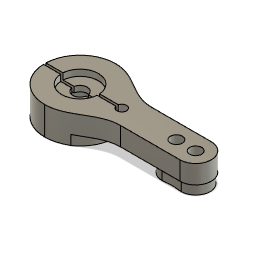
assembled new design (Autodesk Fusion 360 archive; units mm, degrees)
design "servo connector"
Autodesk Fusion 360 part; units mm, degrees
sketch "Sketch1" plane through (0, 0, 0) normal (0, 1, 0) x (1, 0, 0)
  circle A0 centre (0, 0) radius 7.35
  line L0 (0, -3.25) -> (24, -3.25)
  arc A1 (24, -3.25) -> (24, 3.25) centre (24, 0) ccw
  line L1 (24, 3.25) -> (0, 3.25)
  arc A2 (0, 3.25) -> (0, -3.25) centre (0, 0) ccw
  line L2 (0, 0) -> (24, 0) construction
  line L3 (-7.35, 0) -> (11.65, 0) construction
  line L4 (11.65, 0) -> (11.65, 3.25) construction
  circle A3 centre (24, 0) radius 1.25
  circle A4 centre (20, 0) radius 1.25
  spline S0 degree 5 poles (11.65, 3.25) (11.1355, 3.25) (10.1313, 3.3337) (8.6992, 3.7102) (6.9088, 4.6153) (4.7412, 5.9847) (2.9508, 6.8898) (1.5187, 7.2663) (0.5145, 7.35) (0, 7.35) knots 0 0 0 0 0 0 0.2 0.4 0.6 0.8 1 1 1 1 1 1
  line L5 (0, 7.35) -> (0, 0) construction
  spline S1 degree 5 poles (11.65, -3.25) (11.1355, -3.25) (10.1313, -3.3337) (8.6992, -3.7102) (6.9088, -4.6153) (4.7412, -5.9847) (2.9508, -6.8898) (1.5187, -7.2663) (0.5145, -7.35) (0, -7.35) knots 0 0 0 0 0 0 0.2 0.4 0.6 0.8 1 1 1 1 1 1
  line L6 (12.9681, 3.25) -> (10.3319, 3.25)
  line L7 (1.3181, 7.35) -> (-1.3181, 7.35)
  line L8 (12.9681, -3.25) -> (10.3319, -3.25)
  line L9 (1.3181, -7.35) -> (-1.3181, -7.35)
  circle A5 centre (0, 0) radius 1.5
  line L10 (-7.35, 0) -> (8.65, 0) construction
  circle A6 centre (8.65, 0) radius 1
  line L11 (8.65, 0.25) -> (-8, 0.25)
  arc A7 (-8, 0.25) -> (-8, -0.25) centre (-8, 0) ccw
  line L12 (-8, -0.25) -> (8.65, -0.25)
  arc A8 (8.65, -0.25) -> (8.65, 0.25) centre (8.65, 0) ccw
  line L13 (8.65, 0) -> (-8, 0) construction
  dimension "d1" = 14.7
  dimension "d4" = 24
  dimension "d5" = 6.5
  dimension "d6" = 19
  dimension "d7" = 4
  dimension "d8" = 2.5
  dimension "d9" = 2.5
  dimension "d10" = 3
  dimension "d11" = 16
  dimension "d12" = 2
  dimension "d15" = 0.5
  constraint coincident A0.centre A2.centre
  constraint tangent L0 A1
  constraint tangent A1 L1
  constraint parallel L0 L1
  constraint tangent L1 A2
  constraint tangent L0 A2
  constraint horizontal L2
  constraint coincident A0 L3.start
  constraint parallel L2 L3
  constraint coincident L1 L4.end
  constraint perpendicular L1 L4
  constraint concentric A1 A3
  constraint coincident L2 A4.centre
  constraint coincident A0 S0.end
  constraint perpendicular L3 L5
  constraint coincident S0.end L5.start
  constraint tangent A0 S0
  constraint midpoint L4.end L6
  constraint midpoint S0.end L7
  constraint symmetric L3 L4.end S1.start
  constraint symmetric L3 S0.end S1.end
  constraint symmetric L3 L6.start L8.start
  constraint symmetric L3 L6.end L8.end
  constraint symmetric L3 L7.start L9.start
  constraint symmetric L3 L7.end L9.end
  constraint perpendicular L4 L10
  constraint coincident L10.end A6.centre
  constraint tangent L11 A7
  constraint tangent A7 L12
  constraint parallel L11 L12
  constraint tangent L12 A8
  constraint tangent L11 A8
  constraint parallel L3 L13
  measures "d1" diameter of A0
  measures "d4" distance of A0.centre A1.centre
  measures "d5" diameter of A1
  measures "d6" distance of L3.start L3.end
  measures "d7" distance of A1.centre A4.centre
  measures "d8" diameter of A4
  measures "d9" diameter of A3
  measures "d10" diameter of A5
  measures "d11" distance of L3.start L10.end
  measures "d12" diameter of A6
  measures "d15" diameter of A7
extrude "Extrude1" add sketch "Sketch1" along normal blind 5.85 contours A0 L1 A2 A5 L11 | A0 L0 A1 L1 L6 L8 A6 L11 L12 | A0 L0 A2 A5 L12 | A0 L0 A2 L12 | A0 L1 A2 L11 | A0 L1 S0 L6 | A0 L0 S1 L8
sketch "Sketch2" plane through (0, 5.85, 0) normal (0, 1, 0) x (-1, 0, 0)
  circle A0 centre (-20, 0) radius 1.25
  circle A1 centre (-24, 0) radius 1.25
  line L0 (1.479, 0.25) -> (7.3457, 0.25)
  arc A2 (7.3457, 0.25) -> (0, 7.35) centre (0, 0) ccw
  spline S0 degree 5 poles (0, 7.35) (-0.5145, 7.35) (-1.5187, 7.2663) (-2.9508, 6.8898) (-4.7412, 5.9847) (-6.9088, 4.6153) (-8.6992, 3.7102) (-10.1313, 3.3337) (-11.1355, 3.25) (-11.65, 3.25) knots -1 -1 -1 -1 -1 -1 -0.8 -0.6 -0.4 -0.2 0 0 0 0 0 0
  line L1 (-11.65, 3.25) -> (-24, 3.25)
  arc A3 (-24, 3.25) -> (-24, -3.25) centre (-24, 0) ccw
  line L2 (-24, -3.25) -> (-11.65, -3.25)
  spline S1 degree 5 poles (-11.65, -3.25) (-11.1355, -3.25) (-10.1313, -3.3337) (-8.6992, -3.7102) (-6.9088, -4.6153) (-4.7412, -5.9847) (-2.9508, -6.8898) (-1.5187, -7.2663) (-0.5145, -7.35) (0, -7.35) knots 0 0 0 0 0 0 0.2 0.4 0.6 0.8 1 1 1 1 1 1
  arc A4 (0, -7.35) -> (7.3457, -0.25) centre (0, 0) ccw
  line L3 (7.3457, -0.25) -> (1.479, -0.25)
  arc A5 (-1.479, -0.25) -> (1.479, -0.25) centre (0, 0) ccw
  line L4 (-1.479, -0.25) -> (-7.6818, -0.25)
  arc A6 (-7.6818, 0.25) -> (-7.6818, -0.25) centre (-8.65, 0) ccw
  line L5 (-7.6818, 0.25) -> (-1.479, 0.25)
  arc A7 (1.479, 0.25) -> (-1.479, 0.25) centre (0, 0) ccw
  circle A8 centre (0, 0) radius 3.8
  dimension "d16" = 7.6
  constraint concentric A2 A8
  measures "d16" diameter of A8
extrude "Extrude2" cut sketch "Sketch2" against normal blind 1.3 contours L0 L5 A7 A8 | L3 A5 L4 A8
sketch "Sketch3" plane through (0, 0, 0) normal (0, -1, 0) x (1, 0, 0)
  circle A0 centre (20, 0) radius 1.25
  circle A1 centre (24, 0) radius 1.25
  line L0 (-7.3457, 0.25) -> (-1.479, 0.25)
  arc A2 (1.479, 0.25) -> (-1.479, 0.25) centre (0, 0) ccw
  line L1 (1.479, 0.25) -> (7.6818, 0.25)
  arc A3 (7.6818, -0.25) -> (7.6818, 0.25) centre (8.65, 0) ccw
  line L2 (7.6818, -0.25) -> (1.479, -0.25)
  arc A4 (-1.479, -0.25) -> (1.479, -0.25) centre (0, 0) ccw
  line L3 (-1.479, -0.25) -> (-7.3457, -0.25)
  arc A5 (-7.3457, -0.25) -> (0, -7.35) centre (0, 0) ccw
  spline S0 degree 5 poles (11.65, -3.25) (11.1355, -3.25) (10.1313, -3.3337) (8.6992, -3.7102) (6.9088, -4.6153) (4.7412, -5.9847) (2.9508, -6.8898) (1.5187, -7.2663) (0.5145, -7.35) (0, -7.35) knots 0 0 0 0 0 0 0.2 0.4 0.6 0.8 1 1 1 1 1 1
  line L4 (11.65, -3.25) -> (24, -3.25)
  arc A6 (24, -3.25) -> (24, 3.25) centre (24, 0) ccw
  line L5 (24, 3.25) -> (11.65, 3.25)
  spline S1 degree 5 poles (11.65, 3.25) (11.1355, 3.25) (10.1313, 3.3337) (8.6992, 3.7102) (6.9088, 4.6153) (4.7412, 5.9847) (2.9508, 6.8898) (1.5187, 7.2663) (0.5145, 7.35) (0, 7.35) knots 0 0 0 0 0 0 0.2 0.4 0.6 0.8 1 1 1 1 1 1
  arc A7 (0, 7.35) -> (-7.3457, 0.25) centre (0, 0) ccw
  circle A8 centre (0, 0) radius 2.95
  dimension "d19" = 5.9
  constraint concentric A2 A8
  measures "d19" diameter of A8
extrude "Extrude3" cut sketch "Sketch3" against normal blind 3.4 contours L0 A2 L1 A8 | L2 A4 L3 A8
sketch "Sketch4" plane through (0, 0, 0) normal (0, -1, 0) x (1, 0, 0)
  arc A0 (2.9394, 0.25) -> (-2.9394, 0.25) centre (0, 0) ccw
  line L0 (2.9394, 0.25) -> (7.6818, 0.25)
  arc A1 (7.6818, -0.25) -> (7.6818, 0.25) centre (8.65, 0) ccw
  line L1 (7.6818, -0.25) -> (2.9394, -0.25)
  arc A2 (-2.9394, -0.25) -> (2.9394, -0.25) centre (0, 0) ccw
  line L2 (-2.9394, -0.25) -> (-7.3457, -0.25)
  arc A3 (-7.3457, -0.25) -> (0, -7.35) centre (0, 0) ccw
  spline S0 degree 5 poles (11.65, -3.25) (11.1355, -3.25) (10.1313, -3.3337) (8.6992, -3.7102) (6.9088, -4.6153) (4.7412, -5.9847) (2.9508, -6.8898) (1.5187, -7.2663) (0.5145, -7.35) (0, -7.35) knots 0 0 0 0 0 0 0.2 0.4 0.6 0.8 1 1 1 1 1 1
  line L3 (11.65, -3.25) -> (24, -3.25)
  arc A4 (24, -3.25) -> (24, 3.25) centre (24, 0) ccw
  line L4 (24, 3.25) -> (11.65, 3.25)
  spline S1 degree 5 poles (11.65, 3.25) (11.1355, 3.25) (10.1313, 3.3337) (8.6992, 3.7102) (6.9088, 4.6153) (4.7412, 5.9847) (2.9508, 6.8898) (1.5187, 7.2663) (0.5145, 7.35) (0, 7.35) knots 0 0 0 0 0 0 0.2 0.4 0.6 0.8 1 1 1 1 1 1
  arc A5 (0, 7.35) -> (-7.3457, 0.25) centre (0, 0) ccw
  line L5 (-7.3457, 0.25) -> (-2.9394, 0.25)
  circle A6 centre (24, 0) radius 1.25
  circle A7 centre (20, 0) radius 1.25
  circle A8 centre (0, 0) radius 7.5
  circle A9 centre (20, 0) radius 1.25
  circle A10 centre (24, 0) radius 1.25
  circle A11 centre (20, 0) radius 3
  circle A12 centre (24, 0) radius 3
  line L6 (20, 0) -> (20, 3) construction
  line L7 (24, 0) -> (24, 3) construction
  line L8 (22, 2.2361) -> (22, 2.8361) construction
  spline S2 degree 5 poles (20, 3) (20.0835, 3) (20.2496, 2.9967) (20.496, 2.9819) (20.8196, 2.9457) (21.2171, 2.8903) (21.6098, 2.8451) (22, 2.8273) (22.3902, 2.8451) (22.7829, 2.8903) (23.1804, 2.9457) (23.504, 2.9819) (23.7504, 2.9967) (23.9165, 3) (24, 3) knots 0 0 0 0 0 0 0.1 0.2 0.3 0.4 0.5 0.6 0.7 0.8 0.9 1 1 1 1 1 1
  line L9 (20, 0) -> (24, 0) construction
  spline S3 degree 5 poles (20, -3) (20.0835, -3) (20.2496, -2.9967) (20.496, -2.9819) (20.8196, -2.9457) (21.2171, -2.8903) (21.6098, -2.8451) (22, -2.8273) (22.3902, -2.8451) (22.7829, -2.8903) (23.1804, -2.9457) (23.504, -2.9819) (23.7504, -2.9967) (23.9165, -3) (24, -3) knots 0 0 0 0 0 0 0.1 0.2 0.3 0.4 0.5 0.6 0.7 0.8 0.9 1 1 1 1 1 1
  line L10 (19.576, 3) -> (20.424, 3)
  line L11 (23.576, 3) -> (24.424, 3)
  line L12 (19.576, -3) -> (20.424, -3)
  line L13 (23.576, -3) -> (24.424, -3)
  point P0 (22, -2.8361)
  dimension "d22" = 1.75
  dimension "d23" = 1.75
  dimension "d24" = 0.6
  dimension "d27" = 15
  constraint concentric A0 A8
  constraint coincident A7.centre A9.centre
  constraint coincident A11 L6.end
  constraint vertical L6
  constraint coincident A4.centre A6.centre
  constraint coincident A12 L7.end
  constraint vertical L7
  constraint coincident A11 L8.start
  constraint coincident A12 L8.start
  constraint vertical L8
  constraint tangent A11 S2
  constraint tangent A12 S2
  constraint midpoint L6.end L10
  constraint midpoint L7.end L11
  constraint symmetric L6.end L9 S3.start
  constraint symmetric L7.end L9 S3.end
  constraint symmetric L8.end L9 P0
  constraint symmetric L9 L10.start L12.start
  constraint symmetric L9 L10.end L12.end
  constraint symmetric L9 L11.start L13.start
  constraint symmetric L9 L11.end L13.end
  measures "d24" distance of L8.start L8.end
  measures "d27" diameter of A8
extrude "Extrude4" cut sketch "Sketch4" against normal blind 2 contours L0 A1 L1 S0 L3 A4 L4 S1 A8

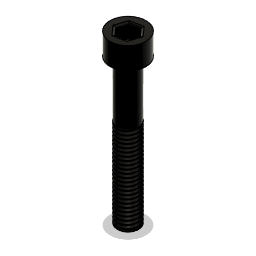
design "M6 45mmm"
Autodesk Fusion 360 part; units mm, degrees
sketch "Sketch1" plane through (0, 0, 0) normal (0, 1, 0) x (1, 0, 0)
  circle A0 centre (0, 0) radius 2.95
  dimension "d1" = 5.9
  constraint coincident A0.centre origin
  measures "d1" diameter of A0
extrude "Extrude1" add sketch "Sketch1" along normal blind 45.5
sketch "Sketch2" plane through (0, 45.5, 0) normal (0, 1, 0) x (-1, 0, 0)
  circle A0 centre (0, 0) radius 2.95
  circle A1 centre (0, 0) radius 4.875
  dimension "d4" = 9.75
  constraint coincident A0.centre A1.centre
  measures "d4" diameter of A1
extrude "Extrude2" add sketch "Sketch2" against normal blind 5.9
sketch "Sketch3" plane through (0, 45.5, 0) normal (0, 1, 0) x (-1, 0, 0)
  circle A0 centre (0, 0) radius 4.875
  line L0 (-2.8282, -0.5783) -> (-0.9133, -2.7385)
  line L1 (-0.9133, -2.7385) -> (1.9149, -2.1602)
  line L2 (1.9149, -2.1602) -> (2.8282, 0.5783)
  line L3 (2.8282, 0.5783) -> (0.9133, 2.7385)
  line L4 (0.9133, 2.7385) -> (-1.9149, 2.1602)
  line L5 (-1.9149, 2.1602) -> (-2.8282, -0.5783)
  dimension "d7" = 2.5
  constraint coincident A0.centre origin
  measures "d7" distance of A0.centre L5
extrude "Extrude3" cut sketch "Sketch3" against normal blind 3.85 contours L0 L1 L2 L3 L4 L5
fillet "Fillet1" radius 0.5 6 edges at (-2.3716, 45.5, -0.791) (-1.8708, 45.5, 1.6584) (0.5008, 45.5, 2.4493) (2.3716, 45.5, 0.791) (1.8708, 45.5, -1.6584) (-0.5008, 45.5, -2.4493)
fillet "Fillet1" radius 0.5 1 edges at (-2.7504, 0, 1.0668)
thread "Thread1" "ISO Metric profile 6.0 M6x1 6g" major diameter 5.884 minor diameter 4.7435 pitch 1 angle 60 modelled right hand crest width 0.1444 on face at (2.9463, 26.5667, 0.147) from (0, 0.5, 0) to (0, 24.5, 0) crest through (2.942, 0.25, 0)
